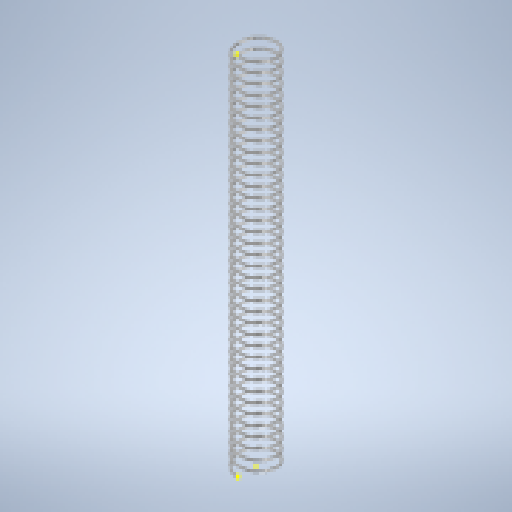
# Autodesk Inventor part: Spring
Saved by Autodesk Inventor 2025.1 (Build 291241020, 241B)
## iProperties
Created: 2024-08-06
Part Number: Spring
Material: Stainless Steel
Document SubType Name: Modeling
Designer: HP-Sourabh
Density: 8 g/cm^3
Appearance: Chrome - Polished
Mass: 19.9599 g
Surface Area: 83.407 cm^2
Volume: 2.49498 cm^3
Author: HP-Sourabh
Autodesk Inventor part; units mm, degrees
ref_plane "YZ Plane" through (0, 0, 0) normal (1, 0, 0) x (0, 1, 0)
ref_plane "XY Plane" through (0, 0, 0) normal (0, 0, 1) x (1, 0, 0)
sketch "Sketch1" plane through (0, 0, 0) normal (1, 0, 0) x (0, 1, 0)
  circle A0 centre (0, 9.4) radius 0.6
  point P0 (0, 0)
  dimension "d0" = 1.2
  dimension "d1" = 9.4
  constraints: 1 centre point, 1 vertical alignment
  measures "d0" diameter of A0
  measures "d1" distance of point (0, 0) A0.centre
coil "Coil1" sketch "Sketch1" operation add axis through (0, -10, 0) along (0, 1, 0) pitch 8 turns 23.75 hand left
sketch "Sketch2" plane through (9.4, 190, 0) normal (0, 0, 1) x (1, 0, 0)
  circle A0 centre (0, 0) radius 0.6 projected
  point P0 (-9.4, -190)
  point P1 (0, 0.6)
  constraints: 1 vertical alignment
ref_plane "Work Plane1" through (9.4, 190, 0) normal (0, 1, 0) x (-1, 0, 0)
sketch "Sketch4" plane through (0, 0, 9.4) normal (1, 0, 0) x (0, 0, -1)
  circle A0 centre (0, 0) radius 0.6 projected
  point P0 (9.4, 0)
  point P1 (0, 0.6)
  constraints: 1 vertical alignment
ref_plane "Work Plane2" through (0, 0, 9.4) normal (0, 1, 0) x (-1, 0, 0)
split "Split1" plane through (9.4, 190, 0) removes the side toward (0, 1, 0)
split "Split2" plane through (0, 0, 9.4) removes the side toward (0, -1, 0)
body "Solid1"
